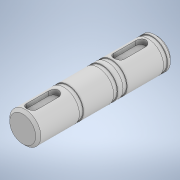
# Autodesk Inventor part: Shaft_stage_input
Saved by Autodesk Inventor 2021 (Build 250183000, 183)
## iProperties
Created: 2020-05-12
Part Number: Shaft_stage_input
Material: Generic
Document SubType Name: Sheet Metal
Designer: avi41
Density: 1 g/cm^3
Appearance: Default
Sheet Metal Rule: Default
Author: avi41
Autodesk Inventor part; units mm, degrees
ref_plane "YZ Plane" through (0, 0, 0) normal (1, 0, 0) x (0, 1, 0)
ref_plane "XY Plane" through (0, 0, 0) normal (0, 0, 1) x (1, 0, 0)
sketch "Sketch1" plane through (0, 0, 0) normal (0, 1, 0) x (-1, 0, 0)
  line L0 (0, -18.13) -> (0, 18.13) construction
  line L1 (-3.6, 0) -> (0.6, 0) construction
  line L2 (0, 12.95) -> (-3, 12.95)
  line L3 (-3, 12.95) -> (-3, -12.95)
  line L4 (-3, -12.95) -> (0, -12.95)
  line L5 (0, 12.95) -> (0, -12.95)
  point P0 (0, 0)
  dimension "d0" = 3
  dimension "d1" = 25.9
  constraints: 8 end point, 3 perpendicular, 2 point on line, 1 horizontal, 1 other
  measures "d0" distance of L3.end L4.end
  measures "d1" distance of L2.end L3.end
revolve "Revolution1" add sketch "Sketch1" angle 360 about axis through (0, 0, 12.95) along (0, 0, -1)
sketch "Sketch2" plane through (0, 0, 0) normal (0, 1, 0) x (-1, 0, 0)
  line L0 (0, -18.2) -> (0, 18.2) construction
  line L1 (-4.2, 0) -> (4.2, 0) construction
  line L2 (-3, 12.95) -> (-3, 12.95)
  line L3 (-3, 4.25) -> (-2.85, 4.25)
  line L4 (-2.85, 4.25) -> (-2.85, 5.05)
  line L5 (-2.85, 5.05) -> (-3, 5.05)
  line L6 (-3, 5.05) -> (-3, 4.25)
  line L7 (-3, 4.25) -> (-3, 5.05)
  line L8 (-3, -12.95) -> (-3, 12.95) projected
  line L9 (3, 12.95) -> (-3, 12.95) projected
  line L10 (-3, -1.55) -> (-2.85, -1.55)
  line L11 (-2.85, -1.55) -> (-2.85, -2.35)
  line L12 (-2.85, -2.35) -> (-3, -2.35)
  line L13 (-3, -2.35) -> (-3, -1.55)
  line L14 (-3, -3.35) -> (-2.85, -3.35)
  line L15 (-2.85, -3.35) -> (-2.85, -4.15)
  line L16 (-2.85, -4.15) -> (-3, -4.15)
  line L17 (-3, -4.15) -> (-3, -3.35)
  line L18 (-3, -11.15) -> (-2.85, -11.15)
  line L19 (-2.85, -11.15) -> (-2.85, -11.95)
  line L20 (-2.85, -11.95) -> (-3, -11.95)
  line L21 (-3, -11.95) -> (-3, -11.15)
  line L22 (3, -12.95) -> (-3, -12.95) projected
  point P0 (-3, -2.35)
  point P1 (-3, -4.15)
  point P2 (-3, -11.95)
  dimension "d34" = 0.8
  dimension "d35" = 2.85
  dimension "d57" = 5.8
  dimension "d58" = 7
  dimension "d59" = 1
  dimension "d63" = 1
  constraints: 36 end point, 8 parallel, 7 collinear, 5 perpendicular, 4 horizontal, 3 point on line
  measures "d34" distance of L3.end L4.end
  measures "d35" distance between parallel lines of L0 L4
  measures "d57" distance between parallel lines of L3 L10
  measures "d58" distance from line of L18 L15.end
  measures "d59" distance between parallel lines of L12 L14
  measures "d63" distance between parallel lines of L20 L22
revolve "Revolution2" cut sketch "Sketch2" angle 360 about axis through (0, 0, 0) along (0, 0, 1)
ref_plane "Work Plane2" through (0, 3, 0) normal (0, 1, 0) x (-1, 0, 0)
sketch "Sketch4" plane through (0, 3, 0) normal (0, 1, 0) x (-1, 0, 0)
  line L0 (0, -26.0074) -> (0, 32.7926) construction
  line L1 (1, -9.725) -> (1, -5.575)
  line L2 (-1, -5.575) -> (-1, -9.725)
  arc A0 (-1, -9.725) -> (1, -9.725) centre (0, -9.725) ccw
  arc A1 (1, -5.575) -> (-1, -5.575) centre (0, -5.575) ccw
  line L3 (3, -12.95) -> (-3, -12.95) projected
  line L4 (-1, -7.65) -> (1, -7.65) construction
  line L5 (-3, -4.15) -> (3, -4.15) construction
  line L6 (3, -11.15) -> (-3, -11.15) construction
  line L7 (0, -17.6074) -> (0, 24.3926) construction
  line L8 (1, 7.05) -> (1, 11.2)
  line L9 (-1, 11.2) -> (-1, 7.05)
  arc A2 (-1, 7.05) -> (1, 7.05) centre (0, 7.05) ccw
  arc A3 (1, 11.2) -> (-1, 11.2) centre (0, 11.2) ccw
  line L10 (3, 12.95) -> (-3, 12.95) projected
  point P0 (0, 0)
  point P1 (1, 1)
  point P2 (0, 24.3926)
  dimension "d49" = 6.15
  dimension "d50" = 1
  dimension "d60" = 3.5
  dimension "d61" = 3.5
  dimension "d64" = 6.15
  dimension "d65" = 1
  dimension "d66" = 1.75
  constraints: 10 end point, 8 point on circle, 6 tangent, 4 centre point, 4 point on line, 3 parallel, 2 midpoint, 6 other
  measures "d50" radius of A0
  measures "d60" distance between parallel lines of L4 L6
  measures "d61" distance between parallel lines of L5 L4
  measures "d65" radius of A2
  measures "d66" distance from line of L10 A3.centre
extrude "Extrusion2" cut sketch "Sketch4" against normal blind 1
chamfer "Chamfer3" distance 0.5 angle 45 2 edges at (-3, 0, -12.95) (-3, 0, 12.95)
equation "\"module\" = 1"
equation "\"pressure_ang\" = 30deg"
equation "\"pitch\" = 3.1416 * module"
equation "\"addendum\" = 0.45 * module"
equation "\"dedendum\" = 0.65 * module"
equation "\"tooth_depth\" = addendum + dedendum"
equation "\"addendum_mod_shaft\" = 0.45 * module"
equation "\"root_fillet_r\" = 0.16 * module"
equation "\"addendum_mod_hub\" = -addendum_mod_shaft"
equation "\"nom_space_t_hub\" = nom_tooth_t_shaft"
equation "\"nom_tooth_t_shaft\" = 2.090415"
body "Solid1"
